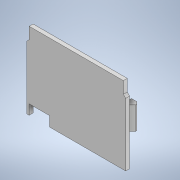
# Autodesk Inventor part: eonPCBcover
Saved by Autodesk Inventor 2020 (Build 240168000, 168)
## iProperties
Created: 2021-04-25
Part Number: eonPCBcover
Material: Generic
Document SubType Name: Modeling
Designer: dkiiv
Density: 1 g/cm^3
Appearance: Default
Author: dkiiv
Autodesk Inventor part; units mm, degrees
ref_plane "YZ Plane" through (0, 0, 0) normal (1, 0, 0) x (0, 1, 0)
ref_plane "XZ Plane" through (0, 0, 0) normal (0, 1, 0) x (-1, 0, 0)
ref_plane "XY Plane" through (0, 0, 0) normal (0, 0, 1) x (1, 0, 0)
sketch "Sketch1" plane through (0, 0, 0) normal (0, 0, 1) x (1, 0, 0)
  line L0 (0, 0) -> (42, 0)
  line L1 (42, 0) -> (42, 26.724)
  line L2 (0, 26.724) -> (0, 26.724)
  line L3 (0, 26.724) -> (0, 0)
  line L4 (1, 26.724) -> (41, 26.724)
  line L5 (41, 27.724) -> (41, 32.724)
  line L6 (41, 32.724) -> (1, 32.724)
  line L7 (1, 32.724) -> (1, 27.724)
  line L8 (1, 27.724) -> (0, 26.724)
  line L9 (42, 26.724) -> (42, 26.724)
  line L10 (41, 27.724) -> (42, 26.724)
  point P0 (42, 26.724)
  dimension "d0" = 26.724
  dimension "d1" = 42
  dimension "d2" = 0
  dimension "d3" = 40
  dimension "d4" = 1
  dimension "d5" = 1
  dimension "d6" = 1
  dimension "d7" = 1
  dimension "d8" = 1
  dimension "d9" = 5
  constraints: 22 end point, 6 point on line, 4 parallel, 2 horizontal, 2 perpendicular
  measures "d0" distance of L2.end L0.start
  measures "d1" distance of L0.start L0.end
  measures "d2" distance between parallel lines of L2 L4
  measures "d3" distance of L5.end L6.end
  measures "d4" distance between parallel lines of L3 L7
  measures "d5" distance of L7.end point (1, 26.724)
  measures "d6" distance of L2.start point (1, 26.724)
  measures "d7" distance of L5.start L4.end
  measures "d8" distance of L9.start L4.end
  measures "d9" distance of L5.start L5.end
extrude "Extrusion1" add sketch "Sketch1" along normal blind 1.667
sketch "Sketch2" plane through (0, 0, 1.667) normal (0, 0, 1) x (1, 0, 0)
  line L0 (32.3, 4.2) -> (41, 4.2)
  line L1 (41, 4.2) -> (41, 0)
  line L2 (41, 0) -> (32.3, 0)
  line L3 (32.3, 0) -> (32.3, 4.2)
  line L4 (0, 0) -> (42, 0) projected
  line L5 (1, 32.724) -> (1, 27.724) projected
  line L6 (41, 27.724) -> (41, 32.724) projected
  dimension "d12" = 0
  dimension "d14" = 8.7
  dimension "d15" = 4.2
  dimension "d18" = 0
  constraints: 8 end point, 2 parallel, 1 horizontal, 1 perpendicular
  measures "d12" distance between parallel lines of L4 L2
  measures "d14" distance of L0.start L0.end
  measures "d15" distance of L0.end L1.end
  measures "d18" distance between parallel lines of L6 L1
extrude "Extrusion2" cut sketch "Sketch2" against normal blind 2.083
sketch "Sketch3" plane through (0, 0, 1.667) normal (0, 0, 1) x (1, 0, 0)
  line L0 (41.75, 13.5) -> (39.75, 13.5)
  line L1 (39.75, 13.5) -> (39.75, 23.2)
  line L2 (39.75, 23.2) -> (41.75, 23.2)
  line L3 (41.75, 23.2) -> (41.75, 13.5)
  line L4 (0.25, 13.5) -> (2.25, 13.5)
  line L5 (2.25, 13.5) -> (2.25, 23.2)
  line L6 (2.25, 23.2) -> (0.25, 23.2)
  line L7 (0.25, 23.2) -> (0.25, 13.5)
  line L8 (0, 0) -> (32.3, 0) projected
  line L9 (0, 26.724) -> (0, 0) projected
  line L10 (42, 0) -> (42, 26.724) projected
  dimension "d19" = 13.5
  dimension "d20" = 0
  dimension "d21" = 23.2
  dimension "d22" = 0
  dimension "d23" = 0.25
  dimension "d24" = 0.25
  dimension "d25" = 2
  dimension "d26" = 2
  constraints: 16 end point, 4 parallel, 2 horizontal, 2 perpendicular
  measures "d19" distance between parallel lines of L8 L4
  measures "d20" distance between parallel lines of L4 L0
  measures "d21" distance between parallel lines of L8 L6
  measures "d22" distance between parallel lines of L2 L6
  measures "d23" distance between parallel lines of L9 L7
  measures "d24" distance between parallel lines of L10 L3
  measures "d25" distance of L5.end L6.end
  measures "d26" distance of L1.end L2.end
extrude "Extrusion3" add sketch "Sketch3" along normal blind 3
sketch "Sketch4" plane through (0.25, 13.5, 1.667) normal (-1, 0, 0) x (0, 0, 1)
  line L0 (0, 9.7) -> (3, 9.7) projected
  line L1 (3, 9.7) -> (1.5, 9.7)
  line L2 (1.5, 9.7) -> (1.5, 0)
  line L3 (1.5, 0) -> (3, 0)
  line L4 (3, 0) -> (3, 9.7)
  line L5 (0, 0) -> (3, 0) projected
  line L6 (0, 13.224) -> (0, -13.5) projected
  point P0 (-1.667, -13.5)
  dimension "d29" = 0
  dimension "d30" = 1.5
  constraints: 8 end point, 2 parallel, 1 horizontal, 1 perpendicular
  measures "d29" distance between parallel lines of L5 L3
  measures "d30" distance between parallel lines of L6 L2
extrude "Extrusion4" add sketch "Sketch4" along normal blind 1.25 contours L0 L4 L3 L2
sketch "Sketch5" plane through (41.75, 13.5, 1.667) normal (1, 0, 0) x (0, 0, -1)
  line L0 (-3, 0) -> (-3, 9.7) projected
  line L1 (-3, 9.7) -> (-1.5, 9.7)
  line L2 (-1.5, 9.7) -> (-1.5, 0)
  line L3 (-1.5, 0) -> (-3, 0)
  line L4 (-3, 0) -> (-3, 9.7)
  line L5 (0, -13.5) -> (0, 13.224) projected
  line L6 (0, 0) -> (-3, 0) projected
  point P0 (1.667, -13.5)
  dimension "d33" = 1.5
  dimension "d34" = 0
  constraints: 8 end point, 2 parallel, 1 horizontal, 1 perpendicular
  measures "d33" distance between parallel lines of L5 L2
  measures "d34" distance between parallel lines of L6 L3
extrude "Extrusion5" add sketch "Sketch5" along normal blind 1.25
chamfer "Chamfer1" distance 1.25 angle 45 2 edges at (41.75, 18.35, 3.167) (0.25, 18.35, 3.167)
sketch "Sketch6" plane through (0, 0, 1.667) normal (0, 0, 1) x (1, 0, 0)
  line L0 (10.3, 2) -> (25.3, 2)
  line L1 (25.3, 2) -> (25.3, 7)
  line L2 (25.3, 7) -> (10.3, 7)
  line L3 (10.3, 7) -> (10.3, 2)
  line L4 (0, 0) -> (32.3, 0) projected
  line L5 (32.3, 0) -> (32.3, 4.2) projected
  dimension "d40" = 2
  dimension "d41" = 15
  dimension "d42" = 5
  dimension "d43" = 7
  constraints: 8 end point, 2 parallel, 1 horizontal, 1 perpendicular
  measures "d40" distance between parallel lines of L4 L0
  measures "d41" distance of L1.end L2.end
  measures "d42" distance of L0.end L1.end
  measures "d43" distance between parallel lines of L5 L1
extrude "Extrusion6" add sketch "Sketch6" along normal blind 10
chamfer "Chamfer2" distance 1 angle 45 2 edges at (43, 18.35, 4.667) (-1, 18.35, 4.667)
fillet "Fillet1" radius 2 2 edges at (39.75, 18.35, 1.667) (2.25, 18.35, 1.667)
equation "\"d6\" = d5"
equation "\"d8\" = d7"
body "Solid1"
